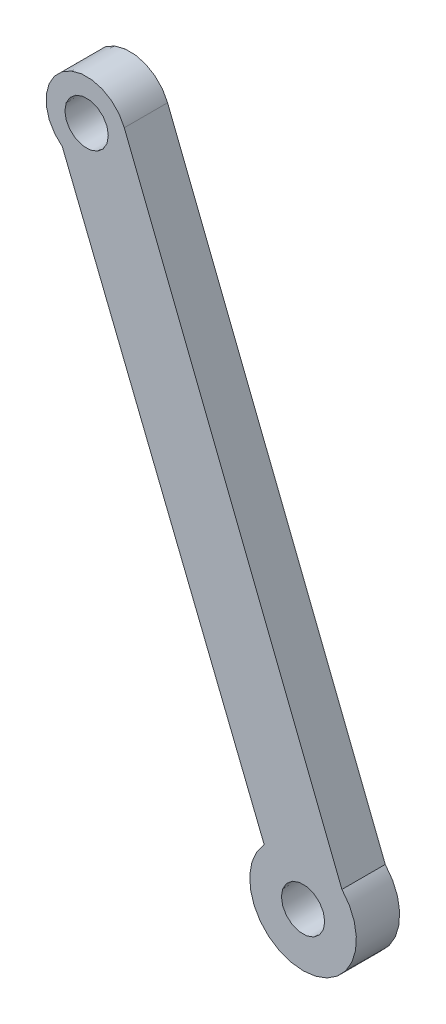
# Autodesk Inventor part: LowerArm
Saved by Autodesk Inventor 2024.1 (Build 281209000, 209)
## iProperties
Created: 2023-08-23
Part Number: LowerArm
Material: Generic
Document SubType Name: Modeling
Designer: Eleanor
Density: 1 g/cm^3
Appearance: Default
Author: Eleanor
Autodesk Inventor part; units mm, degrees
ref_plane "YZ Plane" through (0, 0, 0) normal (1, 0, 0) x (0, 1, 0)
ref_plane "XZ Plane" through (0, 0, 0) normal (0, 1, 0) x (-1, 0, 0)
ref_plane "XY Plane" through (0, 0, 0) normal (0, 0, 1) x (1, 0, 0)
sketch "Sketch5" plane through (0, 0, 0) normal (0, 0, 1) x (1, 0, 0)
  line L0 (8.1925, 0) -> (8.1925, 2.0926)
  point P0 (0, 0)
  constraints: 2 end point, 1 vertical
sketch "Sketch6" plane through (0, 0, 0) normal (0, 0, 1) x (1, 0, 0)
  circle A0 centre (8.1925, 2.0909) radius 1.5875
  point P0 (0, 0)
  dimension "d2" = 3.175
  constraints: 1 centre point
  measures "d2" diameter of A0
sketch "Sketch7" plane through (0, 0, 0) normal (0, 0, 1) x (1, 0, 0)
  circle A0 centre (8.1923, 2.092) radius 1.5921
  circle A1 centre (8.1923, 2.092) radius 2.9715
  circle A2 centre (24.0624, -39.8776) radius 1.5875
  circle A3 centre (24.0624, -39.8776) radius 3.9111
  line L0 (6.4132, -0.2881) -> (21.2107, -37.2008)
  line L1 (26.9141, -37.2008) -> (10.9559, 3.184)
  point P0 (0, 0)
  dimension "d4" = 3.175
  constraints: 4 centre point, 4 end point, 4 point on circle, 2 coincident, 1 tangent
  measures "d4" diameter of A2
extrude "Extrusion1" add sketch "Sketch7" along normal blind 3.175
body "Solid1"
